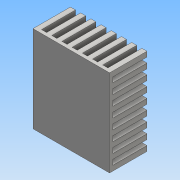
# Autodesk Inventor part: Heat_sink
Saved by Autodesk Inventor 2016 (Build 200138000, 138)
## iProperties
Created: 2016-04-03
Part Number: Heat_sink
Material: Generic
Document SubType Name: Modeling
Designer: admin
Density: 1 g/cm^3
Appearance: Default
Author: admin
Autodesk Inventor part; units mm, degrees
ref_plane "YZ Plane" through (0, 0, 0) normal (1, 0, 0) x (0, 1, 0)
ref_plane "XZ Plane" through (0, 0, 0) normal (0, 1, 0) x (-1, 0, 0)
ref_plane "XY Plane" through (0, 0, 0) normal (0, 0, 1) x (1, 0, 0)
sketch "Sketch1" plane through (0, 0, 0) normal (0, 1, 0) x (-1, 0, 0)
  line L0 (22.5, 25.5) -> (-22.5, 25.5)
  line L1 (-22.5, 25.5) -> (-22.5, -25.5)
  line L2 (-22.5, -25.5) -> (22.5, -25.5)
  line L3 (22.5, -25.5) -> (22.5, 25.5)
  point P0 (0, 0)
  point P1 (0, -25.5)
  point P2 (22.5, 0)
  dimension "d0" = 45
  dimension "d1" = 51
  constraints: 8 end point, 2 midpoint, 2 parallel, 1 horizontal, 1 horizontal alignment, 1 perpendicular, 1 vertical alignment
  measures "d0" distance of L1.end L2.end
  measures "d1" distance of L0.end L1.end
extrude "Extrusion1" add sketch "Sketch1" along normal blind 2
sketch "Sketch2" plane through (0, 2, 0) normal (0, 1, 0) x (1, 0, 0)
  line L0 (-22.5, -25.5) -> (22.5, -25.5) projected
  line L1 (22.5, -25.5) -> (22.5, 25.5) projected
  line L2 (22.5, 25.5) -> (-22.5, 25.5) projected
  line L3 (-22.5, 25.5) -> (-22.5, -25.5) projected
  line L4 (19.5, -25.5) -> (22.5, -25.5)
  line L5 (22.5, -25.5) -> (22.5, -22.5)
  line L6 (22.5, -22.5) -> (19.5, -22.5)
  line L7 (19.5, -22.5) -> (19.5, -25.5)
  line L8 (22.5, -25.5) -> (22.5, 25.5) projected
  line L9 (-22.5, -25.5) -> (22.5, -25.5) projected
  point P0 (0, 0)
  dimension "d4" = 3
  constraints: 8 end point, 2 collinear, 2 parallel, 2 perpendicular, 1 horizontal
  measures "d4" distance of L4.end L5.end
extrude "Extrusion2" add sketch "Sketch2" along normal blind 20 contours L7 L6 L1 L0
pattern_linear "Rectangular Pattern1" count 8 spacing 6 along (-1, 0, 0) count 9 spacing 6 along (0, 0, -1) of "Extrusion2"
body "Solid1"
